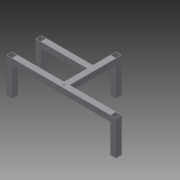
# Autodesk Inventor part: TopSupportV3
Saved by Autodesk Inventor 2013 (Build 170138000, 138)
## iProperties
Created: 2013-08-06
Part Number: TopSupportV3
Material: Generic
Document SubType Name: Modeling
Designer: nowireless
Density: 1 g/cm^3
Author: nowireless
Autodesk Inventor part; units mm, degrees
ref_plane "YZ Plane" through (0, 0, 0) normal (1, 0, 0) x (0, 1, 0)
ref_plane "XZ Plane" through (0, 0, 0) normal (0, 1, 0) x (-1, 0, 0)
ref_plane "XY Plane" through (0, 0, 0) normal (0, 0, 1) x (1, 0, 0)
sketch "Sketch1" plane through (0, 0, 0) normal (1, 0, 0) x (0, 1, 0)
  line L0 (0, 0) -> (25.4, 0)
  line L1 (25.4, 0) -> (25.4, -25.4)
  line L2 (25.4, -25.4) -> (0, -25.4)
  line L3 (0, -25.4) -> (0, 0)
  line L4 (1.5875, -1.5875) -> (23.8125, -1.5875)
  line L5 (23.8125, -1.5875) -> (23.8125, -23.8125)
  line L6 (23.8125, -23.8125) -> (1.5875, -23.8125)
  line L7 (1.5875, -23.8125) -> (1.5875, -1.5875)
  dimension "d0" = 25.4
  dimension "d1" = 1.5875
  dimension "d2" = 1.5875
  dimension "d3" = 1.5875
  dimension "d4" = 1.5875
  constraints: 16 end point, 4 parallel, 4 perpendicular, 2 horizontal
  measures "d0" distance of L0.start L0.end
  measures "d1" distance between parallel lines of L0 L4
  measures "d2" distance between parallel lines of L3 L7
  measures "d3" distance between parallel lines of L2 L6
  measures "d4" distance between parallel lines of L5 L1
extrude "Extrusion1" add sketch "Sketch1" along normal blind 431.8
sketch "Sketch2" plane through (0, 0, -25.4) normal (0, 0, -1) x (-1, 0, 0)
  line L0 (0, 25.4) -> (0, 0) projected
  line L1 (0, 25.4) -> (-431.8, 25.4) projected
  line L2 (0, 0) -> (-431.8, 0) construction
  line L3 (-228.6, 0) -> (-203.2, 0)
  line L4 (-203.2, 0) -> (-203.2, 25.4)
  line L5 (-203.2, 25.4) -> (-228.6, 25.4)
  line L6 (-228.6, 25.4) -> (-228.6, 0)
  line L7 (-215.9, 25.4) -> (-215.9, 0) construction
  line L8 (-227.0125, 1.5875) -> (-204.7875, 1.5875)
  line L9 (-204.7875, 1.5875) -> (-204.7875, 23.8125)
  line L10 (-204.7875, 23.8125) -> (-227.0125, 23.8125)
  line L11 (-227.0125, 23.8125) -> (-227.0125, 1.5875)
  line L12 (-227.0125, 1.5875) -> (-204.7875, 23.8125) construction
  line L13 (-204.7875, 1.5875) -> (-227.0125, 23.8125) construction
  point P0 (-215.9, 12.7)
  dimension "d7" = 25.4
  dimension "d9" = 12.7
  dimension "d10" = 215.9
  dimension "d11" = 1.5875
  dimension "d12" = 1.5875
  dimension "d13" = 1.5875
  dimension "d14" = 1.5875
  constraints: 22 end point, 4 midpoint, 4 parallel, 3 perpendicular, 2 horizontal, 2 point on line
  measures "d7" distance between parallel lines of L4 L6
  measures "d9" distance between parallel lines of L4 L7
  measures "d10" distance between parallel lines of L0 L7
  measures "d11" distance between parallel lines of L1 L10
  measures "d12" distance between parallel lines of L3 L8
  measures "d13" distance between parallel lines of L4 L9
  measures "d14" distance between parallel lines of L6 L11
extrude "Extrusion2" add sketch "Sketch2" along normal blind 203.2
sketch "Sketch3" plane through (203.2, 0, -25.4) normal (-1, 0, 0) x (0, 0, 1)
  line L0 (0, 25.4) -> (0, 0) projected
  line L1 (0, 25.4) -> (-203.2, 25.4) projected
  line L2 (0, 0) -> (-203.2, 0) projected
  line L3 (-127, 0) -> (-101.6, 0)
  line L4 (-101.6, 0) -> (-101.6, 25.4)
  line L5 (-101.6, 25.4) -> (-127, 25.4)
  line L6 (-127, 25.4) -> (-127, 0)
  line L7 (-114.3, 25.4) -> (-114.3, 0) construction
  line L8 (-125.4125, 1.5875) -> (-103.1875, 1.5875)
  line L9 (-103.1875, 1.5875) -> (-103.1875, 23.8125)
  line L10 (-103.1875, 23.8125) -> (-125.4125, 23.8125)
  line L11 (-125.4125, 23.8125) -> (-125.4125, 1.5875)
  point P0 (25.4, 0)
  dimension "d17" = 25.4
  dimension "d19" = 12.7
  dimension "d20" = 114.3
  dimension "d21" = 1.5875
  dimension "d22" = 1.5875
  dimension "d23" = 1.5875
  dimension "d24" = 1.5875
  constraints: 18 end point, 4 parallel, 3 midpoint, 3 perpendicular, 2 horizontal, 1 point on line
  measures "d17" distance between parallel lines of L4 L6
  measures "d19" distance between parallel lines of L4 L7
  measures "d20" distance between parallel lines of L0 L7
  measures "d21" distance between parallel lines of L10 L1
  measures "d22" distance between parallel lines of L4 L9
  measures "d23" distance between parallel lines of L6 L11
  measures "d24" distance between parallel lines of L3 L8
extrude "Extrusion3" add sketch "Sketch3" along normal blind 203.2 contours L4 L2 L6 L1
sketch "Sketch4" plane through (0, 25.4, 0) normal (0, 1, 0) x (1, 0, 0)
  line L0 (0, 0) -> (0, 25.4) projected
  line L1 (431.8, 25.4) -> (431.8, 0) projected
  line L2 (203.2, 228.6) -> (228.6, 228.6) projected
  line L3 (0, 127) -> (-25.4, 127)
  line L4 (-25.4, 127) -> (-25.4, 152.4)
  line L5 (-25.4, 152.4) -> (0, 152.4)
  line L6 (0, 152.4) -> (0, 127)
  line L7 (0, 0) -> (-25.4, 0)
  line L8 (-25.4, 0) -> (-25.4, 25.4)
  line L9 (-25.4, 25.4) -> (0, 25.4)
  line L10 (0, 25.4) -> (0, 0)
  line L11 (431.8, 0) -> (457.2, 0)
  line L12 (457.2, 0) -> (457.2, 25.4)
  line L13 (457.2, 25.4) -> (431.8, 25.4)
  line L14 (431.8, 25.4) -> (431.8, 0)
  line L15 (203.2, 228.6) -> (206.375, 228.6)
  line L16 (-23.8125, 128.5875) -> (-1.5875, 128.5875)
  line L17 (-1.5875, 128.5875) -> (-1.5875, 150.8125)
  line L18 (-1.5875, 150.8125) -> (-23.8125, 150.8125)
  line L19 (-23.8125, 150.8125) -> (-23.8125, 128.5875)
  line L20 (-23.8125, 1.5875) -> (-1.5875, 1.5875)
  line L21 (-1.5875, 1.5875) -> (-1.5875, 23.8125)
  line L22 (-1.5875, 23.8125) -> (-23.8125, 23.8125)
  line L23 (-23.8125, 23.8125) -> (-23.8125, 1.5875)
  line L24 (204.7875, 234.8076) -> (204.7875, 234.8076)
  line L25 (433.3875, 1.5875) -> (455.6125, 1.5875)
  line L26 (455.6125, 1.5875) -> (455.6125, 23.8125)
  line L27 (455.6125, 23.8125) -> (433.3875, 23.8125)
  line L28 (433.3875, 23.8125) -> (433.3875, 1.5875)
  line L29 (203.2, 228.6) -> (228.6, 228.6)
  line L30 (228.6, 228.6) -> (228.6, 254)
  line L31 (228.6, 254) -> (203.2, 254)
  line L32 (203.2, 254) -> (203.2, 228.6)
  line L33 (204.7875, 230.1875) -> (227.0125, 230.1875)
  line L34 (227.0125, 230.1875) -> (227.0125, 252.4125)
  line L35 (227.0125, 252.4125) -> (204.7875, 252.4125)
  line L36 (204.7875, 252.4125) -> (204.7875, 230.1875)
  dimension "d27" = 25.4
  dimension "d28" = 25.4
  dimension "d29" = 25.4
  dimension "d33" = 25.4
  dimension "d34" = 25.4
  dimension "d35" = 1.5875
  dimension "d36" = 1.5875
  dimension "d37" = 1.5875
  dimension "d39" = 1.5875
  dimension "d40" = 1.5875
  dimension "d41" = 1.5875
  dimension "d42" = 1.5875
  dimension "d43" = 1.5875
  dimension "d44" = 1.5875
  dimension "d45" = 1.5875
  dimension "d46" = 1.5875
  dimension "d47" = 1.5875
  dimension "d48" = 1.5875
  dimension "d49" = 1.5875
  dimension "d50" = 1.5875
  dimension "d51" = 1.5875
  constraints: 68 end point, 16 parallel, 10 horizontal, 8 perpendicular
  measures "d27" distance of L3.start L3.end
  measures "d28" distance of L0.start L7.end
  measures "d29" distance of L1.end L11.end
  measures "d33" distance of L29.end L30.end
  measures "d34" distance of L30.end L31.end
  measures "d35" distance between parallel lines of L31 L35
  measures "d36" distance between parallel lines of L30 L34
  measures "d37" distance between parallel lines of L32 L36
  measures "d39" distance between parallel lines of L2 L33
  measures "d40" distance between parallel lines of L18 L5
  measures "d41" distance between parallel lines of L4 L19
  measures "d42" distance between parallel lines of L6 L17
  measures "d43" distance between parallel lines of L3 L16
  measures "d44" distance between parallel lines of L8 L23
  measures "d45" distance between parallel lines of L7 L20
  measures "d46" distance between parallel lines of L0 L21
  measures "d47" distance between parallel lines of L22 L9
  measures "d48" distance between parallel lines of L1 L28
  measures "d49" distance between parallel lines of L12 L26
  measures "d50" distance between parallel lines of L13 L27
  measures "d51" distance between parallel lines of L11 L25
extrude "Extrusion4" add sketch "Sketch4" against normal blind 152.4
sketch "Sketch5" plane through (203.2, 25.4, -25.4) normal (0, 1, 0) x (1, 0, 0)
  line L0 (-228.6, -25.4) -> (254, -25.4) projected
  line L1 (228.6, -23.8125) -> (228.6, -1.5875) projected
  point P0 (-203.2, -25.4)
  point P1 (12.7, -12.7)
  dimension "d54" = 12.7
  dimension "d55" = 215.9
  measures "d54" distance from line of L0 point (12.7, -12.7)
  measures "d55" distance from line of L1 point (12.7, -12.7)
hole "Hole1" at (215.9, 25.4, -12.7) direction (0, -1, 0) diameter 6.35 depth 25.4 tip angle 118
body "Solid1"
